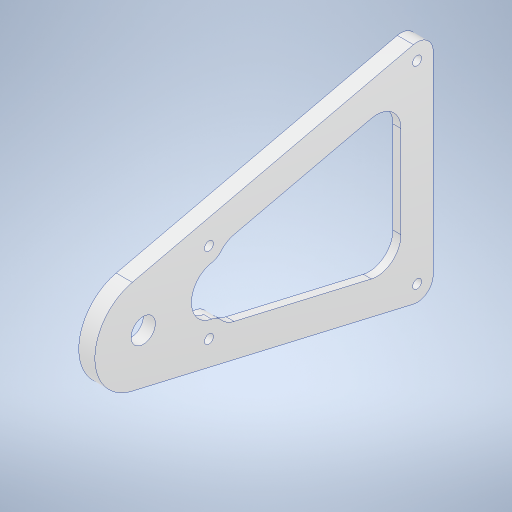
# Autodesk Inventor part: Frame (Motor Side)
Saved by Autodesk Inventor 2023.2 (Build 272271000, 271)
## iProperties
Created: 2022-05-22
Part Number: Frame (Motor Side)
Material: Aluminum 6061
Document SubType Name: Modeling
Designer: Nathan Cai
Density: 2.7 g/cm^3
Appearance: Aluminum - Flat
Mass: 63.0203 g
Surface Area: 136.097 cm^2
Volume: 23.3409 cm^3
Leg_Mounts: 0.625 in
Leg_Offset: 0.750 in
C2C: 4.250 in
Author: Nathan Cai
Autodesk Inventor part; units mm, degrees
ref_plane "YZ Plane" through (0, 0, 0) normal (1, 0, 0) x (0, 1, 0)
ref_plane "XZ Plane" through (0, 0, 0) normal (0, 1, 0) x (-1, 0, 0)
ref_plane "XY Plane" through (0, 0, 0) normal (0, 0, 1) x (1, 0, 0)
sketch "Sketch1" plane through (0, 0, 0) normal (1, 0, 0) x (0, 1, 0)
  circle A0 centre (0, 0) radius 4.7625 construction
  line L0 (0, 0) -> (0, 107.95) construction
  circle A1 centre (0, 107.95) radius 4.7625
  circle A2 centre (0, 107.95) radius 76.2 construction
  circle A3 centre (0, 107.95) radius 19.05
  line L1 (0, 0) -> (38.1, 0) construction
  circle A4 centre (38.1, 0) radius 1.7526
  circle A5 centre (38.1, 0) radius 6.35
  line L2 (18.5565, 112.2582) -> (44.2855, 1.4361)
  line L3 (10.2473, 91.8909) -> (31.9145, -1.4361)
  circle A6 centre (-38.1, 0) radius 1.7526
  circle A7 centre (-38.1, 0) radius 6.35
  line L4 (-18.5565, 112.2582) -> (-44.2855, 1.4361)
  line L5 (-10.2473, 91.8909) -> (-31.9145, -1.4361)
  line L6 (38.1, 6.35) -> (-38.1, 6.35)
  line L7 (-38.1, -6.35) -> (38.1, -6.35)
  line L8 (38.1, 0) -> (15.5821, 96.9909) construction
  circle A8 centre (19.05, 82.0537) radius 1.7526
  circle A9 centre (-19.05, 82.0537) radius 1.7526
  line L9 (19.05, 82.0537) -> (-19.05, 82.0537) construction
  circle A10 centre (15.875, 82.0537) radius 6.35
  circle A11 centre (15.875, 82.0537) radius 1.7526
  circle A12 centre (-15.875, 82.0537) radius 6.35
  circle A13 centre (-15.875, 82.0537) radius 1.7526
  arc A14 (31.7424, -0.6947) -> (-31.1085, -6.35) centre (0, 0) ccw construction
  arc A15 (44.45, 0) -> (-44.45, 0) centre (0, 0) ccw construction
  point P0 (44.2067, -1.741)
  point P1 (-22.5238, 39.0123)
  point P2 (-10.2473, 91.8909)
  point P3 (30.1069, 6.35)
  point P4 (-30.1069, 6.35)
  point P5 (-13.9349, 76.0073)
  point P6 (-11.4694, 86.6268)
  point P7 (11.4694, 86.6268)
  point P8 (13.9349, 76.0073)
  point P9 (22.7099, 38.2108)
  point P10 (-22.7099, 38.2108)
  point P11 (-40.2302, 18.9032)
  point P12 (-44.3636, 7.3939)
  point P13 (-31.75, 0)
  point P14 (31.75, 0)
  point P15 (44.3636, 7.3939)
  point P16 (40.2302, 18.9032)
  point P17 (-28.1895, 14.6088)
  point P18 (31.8736, 5.0775)
  point P19 (-31.7424, -0.6947)
  point P20 (28.1895, 14.6088)
  dimension "d0" = 9.525
  dimension "C2C" = 107.95
  dimension "d3" = 9.525
  dimension "d4" = 152.4
  dimension "d5" = 38.1
  dimension "d6" = 38.1
  dimension "d7" = 3.5052
  dimension "d8" = 12.7
  dimension "d9" = 0
  dimension "d10" = 12.7
  dimension "d37" = 3.5052
  dimension "Leg_Offset" = 19.05
  dimension "d39" = 12.7
  dimension "d40" = 3.5052
  dimension "Leg_Mounts" = 15.875
  dimension "d42" = 12.7
  constraints: 20 end point, 18 point on circle, 16 centre point, 11 coincident, 10 symmetric about line, 7 tangent, 6 point on line, 2 horizontal, 2 parallel, 1 vertical, 5 other
  measures "d0" diameter of A0
  measures "C2C" distance of L0.start L0.end
  measures "d3" diameter of A1
  measures "d4" diameter of A2
  measures "d5" diameter of A3
  measures "d6" distance of L1.start L1.end
  measures "d7" diameter of A4
  measures "d8" diameter of A5
  measures "d9" distance from line of A0.centre L1
  measures "d10" distance between parallel lines of L2 L3
  measures "d37" diameter of A8
  measures "Leg_Offset" distance from line of L0 L9.start
  measures "d39" diameter of A10
  measures "d40" diameter of A11
  measures "Leg_Mounts" distance from line of L0 A11.centre
  measures "d42" radial gap between concentric circles of A14 A15
extrude "Extrusion1" add sketch "Sketch1" along normal blind 6.35 contours A3 | A3 L2 A5 L6 L3 A10 | A3 L5 A12 L6 A7 L4 | A5 | A10 L3 | L3 A10 | A7 | A5 L3 L6 | A12 L5 | L5 A12 | L6 L5 A7 | A7 L5 L6 L3 A5 L7 | A8 A11 | A13 A9 picked at (19.7267, 81.9115) picked at (-19.7267, 82.1959)
fillet "Fillet1" radius 9.525 8 edges at (3.175, 10.2473, 91.8909) (3.175, -10.2473, 91.8909) (3.175, 13.9349, 76.0073) (3.175, -13.9349, 76.0073) (3.175, 11.4694, 86.6268) (3.175, -11.4694, 86.6268) (3.175, 30.1069, 6.35) (3.175, -30.1069, 6.35)
sketch "Sketch2" plane through (0, 0, 0) normal (1, 0, 0) x (0, 0, -1)
  circle A0 centre (-107.95, 0) radius 11.1125
  arc A1 (-73.5827, 21.0167) -> (-82.0537, 15.875) centre (-69.9925, 5.553) ccw
  arc A2 (-82.0537, 15.875) -> (-95.2504, 0.1011) centre (-79.3759, 0.2275) ccw
  arc A3 (-95.2504, -0.1011) -> (-95.2504, 0.1011) centre (-107.95, 0) ccw
  arc A4 (-95.2504, -0.1011) -> (-82.0537, -15.875) centre (-79.3759, -0.2275) ccw
  arc A5 (-82.0537, -15.875) -> (-73.5827, -21.0167) centre (-69.9925, -5.553) ccw
  line L0 (-73.5827, -21.0167) -> (-6.1855, -36.6639)
  line L1 (-6.1855, 36.6639) -> (-73.5827, 21.0167)
  circle A6 centre (-82.0537, 15.875) radius 1.7526 projected
  arc A7 (-80.9826, 9.616) -> (-77.2292, 11.7462) centre (-82.0537, 15.875) ccw projected
  circle A8 centre (-82.0537, 15.875) radius 6.35
  circle A9 centre (-82.0537, -15.875) radius 1.7526 projected
  arc A10 (-77.2292, -11.7462) -> (-80.9826, -9.616) centre (-82.0537, -15.875) ccw projected
  circle A11 centre (-82.0537, -15.875) radius 6.35
  line L2 (-1.4361, 44.2855) -> (-112.2582, 18.5565) projected
  circle A12 centre (0, 38.1) radius 6.35
  circle A13 centre (0, -38.1) radius 1.7526 projected
  arc A14 (-1.4361, -44.2855) -> (6.35, -38.1) centre (0, -38.1) ccw projected
  circle A15 centre (0, -38.1) radius 6.35
  circle A16 centre (0, 38.1) radius 1.7526 projected
  line L3 (0, 38.1) -> (0, -38.1)
  arc A17 (-72.1466, 14.8312) -> (-77.2292, 11.7462) centre (-69.9925, 5.553) ccw projected
  line L4 (-72.1466, 14.8312) -> (-18.0291, 27.3954) projected
  arc A18 (-6.35, 18.1172) -> (-18.0291, 27.3954) centre (-15.875, 18.1172) ccw projected
  line L5 (-6.35, 18.1172) -> (-6.35, -18.1172) projected
  arc A19 (-18.0291, -27.3954) -> (-6.35, -18.1172) centre (-15.875, -18.1172) ccw projected
  line L6 (-18.0291, -27.3954) -> (-72.1466, -14.8312) projected
  arc A20 (-77.2292, -11.7462) -> (-72.1466, -14.8312) centre (-69.9925, -5.553) ccw projected
  arc A21 (-77.2292, -11.7462) -> (-80.9826, -9.616) centre (-82.0537, -15.875) ccw projected
  arc A22 (-88.9006, -0.1516) -> (-80.9826, -9.616) centre (-79.3759, -0.2275) ccw projected
  arc A23 (-88.9006, -0.1516) -> (-88.9006, 0.1516) centre (-107.95, 0) ccw projected
  arc A24 (-80.9826, 9.616) -> (-88.9006, 0.1516) centre (-79.3759, 0.2275) ccw projected
  arc A25 (-80.9826, 9.616) -> (-77.2292, 11.7462) centre (-82.0537, 15.875) ccw projected
  circle A26 centre (0, -38.1) radius 1.7526 projected
  circle A27 centre (-82.0537, -15.875) radius 1.7526 projected
  circle A28 centre (-107.95, 0) radius 4.7625 projected
  circle A29 centre (-82.0537, 15.875) radius 1.7526 projected
  circle A30 centre (0, 38.1) radius 1.7526 projected
  line L7 (6.35, -38.1) -> (6.35, 38.1) projected
  arc A31 (6.35, 38.1) -> (-1.4361, 44.2855) centre (0, 38.1) ccw projected
  line L8 (-1.4361, 44.2855) -> (-112.2582, 18.5565) projected
  arc A32 (-112.2582, 18.5565) -> (-112.2582, -18.5565) centre (-107.95, 0) ccw projected
  line L9 (-112.2582, -18.5565) -> (-1.4361, -44.2855) projected
  arc A33 (-1.4361, -44.2855) -> (6.35, -38.1) centre (0, -38.1) ccw projected
  arc A34 (-72.1466, 14.8312) -> (-77.2292, 11.7462) centre (-69.9925, 5.553) ccw projected
  line L10 (-72.1466, 14.8312) -> (-18.0291, 27.3954) projected
  arc A35 (-6.35, 18.1172) -> (-18.0291, 27.3954) centre (-15.875, 18.1172) ccw projected
  line L11 (-6.35, 18.1172) -> (-6.35, -18.1172) projected
  arc A36 (-18.0291, -27.3954) -> (-6.35, -18.1172) centre (-15.875, -18.1172) ccw projected
  line L12 (-18.0291, -27.3954) -> (-72.1466, -14.8312) projected
  arc A37 (-77.2292, -11.7462) -> (-72.1466, -14.8312) centre (-69.9925, -5.553) ccw projected
  arc A38 (-77.2292, -11.7462) -> (-80.9826, -9.616) centre (-82.0537, -15.875) ccw projected
  arc A39 (-88.9006, -0.1516) -> (-80.9826, -9.616) centre (-79.3759, -0.2275) ccw projected
  arc A40 (-88.9006, -0.1516) -> (-88.9006, 0.1516) centre (-107.95, 0) ccw projected
  arc A41 (-80.9826, 9.616) -> (-88.9006, 0.1516) centre (-79.3759, 0.2275) ccw projected
  arc A42 (-80.9826, 9.616) -> (-77.2292, 11.7462) centre (-82.0537, 15.875) ccw projected
  circle A43 centre (0, -38.1) radius 1.7526 projected
  circle A44 centre (-82.0537, -15.875) radius 1.7526 projected
  circle A45 centre (-107.95, 0) radius 4.7625 projected
  circle A46 centre (-82.0537, 15.875) radius 1.7526 projected
  circle A47 centre (0, 38.1) radius 1.7526 projected
  line L13 (6.35, -38.1) -> (6.35, 38.1) projected
  arc A48 (6.35, 38.1) -> (-1.4361, 44.2855) centre (0, 38.1) ccw projected
  line L14 (-1.4361, 44.2855) -> (-112.2582, 18.5565) projected
  arc A49 (-112.2582, 18.5565) -> (-112.2582, -18.5565) centre (-107.95, 0) ccw projected
  line L15 (-112.2582, -18.5565) -> (-1.4361, -44.2855) projected
  arc A50 (-1.4361, -44.2855) -> (6.35, -38.1) centre (0, -38.1) ccw projected
  line L16 (-18.0291, -27.3954) -> (-72.1466, -14.8312) projected
  point P0 (0, 0)
  point P1 (-87.972, 13.5737)
  point P2 (-87.972, -13.5737)
  point P3 (-77.0434, -19.7762)
  point P4 (0, -31.75)
  point P5 (0, 31.75)
  point P6 (-77.0434, 19.7762)
  point P7 (-80.9826, -9.616)
  point P8 (-80.9826, 9.616)
  point P9 (6.35, -38.1)
  point P10 (6.35, 38.1)
  dimension "d44" = 22.225
  dimension "d53" = 6.35
  dimension "d55" = 6.35
  dimension "d56" = 6.35
  dimension "d57" = 6.35
  dimension "d58" = 6.35
  dimension "d59" = 6.35
  dimension "d60" = 6.35
  constraints: 14 point on circle, 8 centre point, 6 end point, 5 coincident, 1 parallel, 1 vertical, 6 other
  measures "d44" diameter of A0
  measures "d53" distance between parallel lines of L4 L1
  measures "d55" distance between parallel lines of L12 L0
  measures "d56" radial gap between concentric circles of A17 A1
  measures "d57" radial gap between concentric circles of A20 A5
  measures "d58" radial gap between concentric circles of A22 A4
  measures "d59" radial gap between concentric circles of A24 A2
  measures "d60" radial gap between concentric circles of A23 A3
extrude "Extrusion4" cut sketch "Sketch2" along normal blind 3.175 contours L1 A12 L3 A15 L0 A5 A11 A20 L6 A19 L5 A18 L4 A17 A8 A1 | A8 A24 A23 A22 A11 A4 A3 A2 | A12 L7 A15 L3
extrude "Extrusion5" cut sketch "Sketch2" along normal blind 1.5875 contours A0 | A28
fillet "Fillet4" radius 6.35 6 edges at (1.5875, 13.5737, 87.972) (1.5875, -13.5737, 87.972) (1.5875, 19.7762, 77.0434) (1.5875, -19.7762, 77.0434) (1.5875, 36.6639, 6.1855) (1.5875, -36.6639, 6.1855)
equation "\"d10\" = d8"
body "Solid1"
